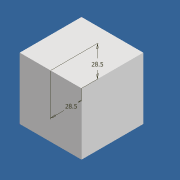
# Autodesk Inventor part: Cube
Saved by Autodesk Inventor 2020 (Build 240168000, 168)
## iProperties
Created: 2019-12-14
Part Number: Cube
Material: Generic
Document SubType Name: Modeling
Designer: Jack
Density: 1 g/cm^3
Appearance: Default
Author: Jack
Autodesk Inventor part; units mm, degrees
ref_plane "YZ Plane" through (0, 0, 0) normal (1, 0, 0) x (0, 1, 0)
ref_plane "XZ Plane" through (0, 0, 0) normal (0, 1, 0) x (-1, 0, 0)
ref_plane "XY Plane" through (0, 0, 0) normal (0, 0, 1) x (1, 0, 0)
sketch "Sketch1" plane through (0, 0, 0) normal (0, 1, 0) x (-1, 0, 0)
  line L0 (-28.5, 28.5) -> (28.5, 28.5)
  line L1 (28.5, 28.5) -> (28.5, -28.5)
  line L2 (28.5, -28.5) -> (-28.5, -28.5)
  line L3 (-28.5, -28.5) -> (-28.5, 28.5)
  line L4 (-28.5, 28.5) -> (28.5, -28.5) construction
  line L5 (28.5, 28.5) -> (-28.5, -28.5) construction
  point P0 (0, 0)
  dimension "d0" = 57
  dimension "d1" = 57
  constraints: 12 end point, 2 midpoint, 2 parallel, 1 horizontal, 1 perpendicular
  measures "d0" distance of L1.end L2.end
  measures "d1" distance of L0.end L1.end
extrude "Extrusion1" add sketch "Sketch1" along normal blind 57
sketch "Sketch2" plane through (0, 0, 0) normal (0, -1, 0) x (1, 0, 0)
  point P0 (0, 0)
sketch "Sketch3" plane through (-28.5, 0, -28.5) normal (-1, 0, 0) x (0, 0, 1)
  line L0 (0, 0) -> (0, 57) projected
  line L1 (0, 0) -> (57, 0) projected
  circle A0 centre (28.5, 28.5) radius 4
  point P0 (28.5, 0)
  dimension "d6" = 8
  dimension "d7" = 28.5
  dimension "d8" = 28.5
  constraints: 1 centre point, 1 coincident
  measures "d6" diameter of A0
  measures "d7" distance from line of L0 point (28.5, 28.5)
  measures "d8" distance from line of L1 point (28.5, 28.5)
sketch "Sketch4" plane through (-28.5, 0, -28.5) normal (-1, 0, 0) x (0, 0, 1)
  line L0 (57, 19) -> (0, 19)
  line L1 (57, 0) -> (57, 57) projected
  line L2 (0, 0) -> (0, 57) projected
  line L3 (57, 38) -> (0, 38)
  line L4 (0, 0) -> (57, 0) projected
  point P0 (28.5, 0)
  dimension "d9" = 19
  dimension "d10" = 19
  constraints: 4 end point, 4 point on line, 2 horizontal
  measures "d9" distance between parallel lines of L4 L0
  measures "d10" distance between parallel lines of L0 L3
equation "\"d10\" = d9"
body "Solid1"
